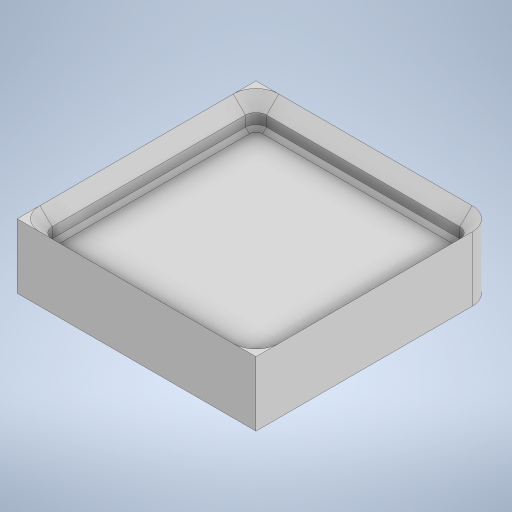
# Autodesk Inventor part: base-plate-weighted
Saved by Autodesk Inventor 2023 (Build 270158030, 158C)
## iProperties
Created: 2023-12-22
Part Number: base-plate-weighted
Material: Generic
Document SubType Name: Modeling
Designer: Imogen Heard
Density: 1 g/cm^3
Appearance: Default
Author: Imogen Heard
Autodesk Inventor part; units mm, degrees
ref_plane "YZ Plane" through (0, 0, 0) normal (1, 0, 0) x (0, 1, 0)
ref_plane "XZ Plane" through (0, 0, 0) normal (0, 1, 0) x (-1, 0, 0)
ref_plane "XY Plane" through (0, 0, 0) normal (0, 0, 1) x (1, 0, 0)
sketch "Sketch1" plane through (0, 0, 0) normal (0, 1, 0) x (-1, 0, 0)
  line L0 (0, -42) -> (-38, -42)
  line L1 (-42, -38) -> (-42, 0)
  line L2 (-42, 0) -> (0, 0)
  line L3 (0, 0) -> (0, -42)
  arc A0 (-42, -38) -> (-38, -42) centre (-38, -38) ccw
  point P0 (-42, -42)
  dimension "d0" = 42
  dimension "d1" = 42
  dimension "d31" = 4
  constraints: 8 end point, 2 parallel, 2 point on circle, 2 point on line, 2 tangent, 1 centre point, 1 coincident, 1 horizontal, 1 perpendicular
  measures "d0" distance between parallel lines of L1 L3
  measures "d1" distance between parallel lines of L2 L0
  measures "d31" radius of A0
extrude "square-base" add sketch "Sketch1" along normal blind 4.65
sketch "Sketch2" plane through (0, 4.65, 0) normal (0, 1, 0) x (1, 0, 0)
  line L0 (4, 39.15) -> (38, 39.15)
  line L1 (39.15, 38) -> (39.15, 4)
  line L2 (38, 2.85) -> (4, 2.85)
  line L3 (2.85, 4) -> (2.85, 38)
  line L4 (38, 42) -> (0, 42) projected
  line L5 (0, 42) -> (0, 0) projected
  line L6 (42, 0) -> (42, 38) projected
  line L7 (0, 0) -> (42, 0) projected
  arc A0 (39.15, 38) -> (38, 39.15) centre (38, 38) ccw
  arc A1 (38, 2.85) -> (39.15, 4) centre (38, 4) ccw
  arc A2 (2.85, 4) -> (4, 2.85) centre (4, 4) ccw
  arc A3 (4, 39.15) -> (2.85, 38) centre (4, 38) ccw
  point P0 (2.85, 39.15)
  point P1 (39.15, 2.85)
  point P2 (39.15, 39.15)
  point P3 (2.85, 2.85)
  point P4 (42, 42)
  dimension "d4" = 2.85
  dimension "d5" = 2.85
  dimension "d6" = 2.85
  dimension "d7" = 2.85
  dimension "d29" = 1.15
  constraints: 8 end point, 8 point on circle, 8 point on line, 8 tangent, 4 centre point, 3 equal radius, 2 parallel, 1 horizontal, 1 perpendicular
  measures "d4" distance between parallel lines of L4 L0
  measures "d5" distance between parallel lines of L5 L3
  measures "d6" distance between parallel lines of L6 L1
  measures "d7" distance between parallel lines of L7 L2
  measures "d29" radius of A0
extrude "Extrusion2" cut sketch "Sketch2" against normal through all
sketch "Sketch3" plane through (0, 4.65, 0) normal (0, 1, 0) x (1, 0, 0)
  line L0 (38, 2.15) -> (4, 2.15)
  line L1 (2.15, 4) -> (2.15, 38)
  line L2 (4, 39.85) -> (38, 39.85)
  line L3 (39.85, 38) -> (39.85, 4)
  line L4 (0, 42) -> (0, 0) projected
  line L5 (38, 2.85) -> (4, 2.85) projected
  line L6 (42, 0) -> (42, 38) projected
  line L7 (38, 42) -> (0, 42) projected
  line L8 (0, 0) -> (42, 0) projected
  line L9 (39.15, 38) -> (39.15, 4) projected
  line L10 (2.85, 4) -> (2.85, 38) projected
  line L11 (4, 39.15) -> (38, 39.15) projected
  arc A0 (39.85, 38) -> (38, 39.85) centre (38, 38) ccw
  arc A1 (38, 2.15) -> (39.85, 4) centre (38, 4) ccw
  arc A2 (2.15, 4) -> (4, 2.15) centre (4, 4) ccw
  arc A3 (4, 39.85) -> (2.15, 38) centre (4, 38) ccw
  point P0 (39.85, 2.15)
  point P1 (2.15, 39.85)
  point P2 (2.15, 2.15)
  point P3 (39.85, 39.85)
  point P4 (39.15, 2.85)
  point P5 (2.85, 2.85)
  point P6 (42, 42)
  point P7 (39.15, 39.15)
  point P8 (2.85, 39.15)
  dimension "d10" = 2.15
  dimension "d12" = 2.15
  dimension "d13" = 2.15
  dimension "d14" = 2.15
  dimension "d30" = 1.85
  constraints: 8 end point, 8 point on circle, 8 point on line, 8 tangent, 4 centre point, 3 equal radius, 2 parallel, 1 horizontal, 1 perpendicular
  measures "d10" distance between parallel lines of L4 L1
  measures "d12" distance between parallel lines of L6 L3
  measures "d13" distance between parallel lines of L7 L2
  measures "d14" distance between parallel lines of L8 L0
  measures "d30" radius of A0
extrude "Extrusion3" cut sketch "Sketch3" against normal blind 3.95
chamfer "Chamfer2" distance 0.7 angle 45 4 edges at (39.15, 0.7, -21) (21, 0.7, -2.85) (2.85, 0.7, -21) (21, 0.7, -39.15)
chamfer "Chamfer1" distance 2.15 angle 45 8 edges at (39.85, 4.65, -21) (39.3081, 4.65, -2.6919) (21, 4.65, -2.15) (2.6919, 4.65, -2.6919) (2.15, 4.65, -21) (2.6919, 4.65, -39.3081) (21, 4.65, -39.85) (39.3081, 4.65, -39.3081)
sketch "Sketch5" plane through (0, 0, 0) normal (0, -1, 0) x (1, 0, 0)
  arc A0 (38, -39.15) -> (39.15, -38) centre (38, -38) ccw projected
  line L0 (38, -39.15) -> (4, -39.15) projected
  arc A1 (2.85, -38) -> (4, -39.15) centre (4, -38) ccw projected
  line L1 (2.85, -38) -> (2.85, -4) projected
  arc A2 (4, -2.85) -> (2.85, -4) centre (4, -4) ccw projected
  line L2 (4, -2.85) -> (38, -2.85) projected
  arc A3 (39.15, -4) -> (38, -2.85) centre (38, -4) ccw projected
  line L3 (39.15, -4) -> (39.15, -38) projected
  line L4 (38, -42) -> (0, -42) projected
  arc A4 (38, -42) -> (42, -38) centre (38, -38) ccw projected
  line L5 (42, 0) -> (42, -38) projected
  line L6 (0, 0) -> (42, 0) projected
  line L7 (0, -42) -> (0, 0) projected
extrude "weighted-base" add sketch "Sketch5" along normal blind 6.7 contours L0 A1 L1 A2 L2 A3 L3 A0 | L4 L7 L6 L5 A4
equation "\"d1\" = d0"
equation "\"d5\" = d4"
equation "\"d6\" = d4"
equation "\"d7\" = d4"
equation "\"d12\" = d10"
equation "\"d13\" = d10"
equation "\"d14\" = d10"
body "Solid1"
